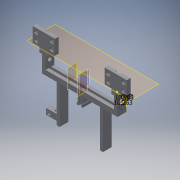
# Autodesk Inventor part: frontChassis_final
Saved by Autodesk Inventor 2018 (Build 220112000, 112)
## iProperties
Created: 2017-10-21
Part Number: frontChassis_final
Material: Generic
Document SubType Name: Modeling
Designer: Prakash
Density: 1 g/cm^3
Appearance: Default
d0: 1.500 mm
d1: 10.000 mm
d2: 18.000 mm
d3: 18.000 mm
d4: 30.000 mm
d5: 0.00 deg
d8: 10.000 mm
d9: 0.00 deg
d10: 3.588 mm
d11: 3.588 mm
d12: 34.763 mm
d13: 0.00 deg
d15: 9.763 mm
d16: 9.525 mm
d17: 8.000 mm
d19: 0.00 deg
d20: 4.000 mm
d21: 0.00 deg
d22: 10.000 mm
d25: 10.000 mm
d26: 5.000 mm
d27: 70.000 mm
d28: 0.00 deg
d74: 7.000 mm
d75: 7.000 mm
d76: 7.500 mm
d77: 7.500 mm
d79: 7.500 mm
d80: 7.500 mm
d81: 3.500 mm
d89: 8.000 mm
d90: 3.175 mm
d91: 0.00 deg
d104: -68.000 mm
d106: 19.526 mm
d107: 9.526 mm
d108: 8.000 mm
d112: 25.000 mm
d113: 7.175 mm
d114: 0.00 deg
d115: 4.000 mm
d116: 0.00 deg
d117: 45.250 mm
Author: Prakash
Autodesk Inventor part; units mm, degrees
ref_plane "YZ Plane" through (0, 0, 0) normal (1, 0, 0) x (0, 1, 0)
ref_plane "XZ Plane" through (0, 0, 0) normal (0, 1, 0) x (-1, 0, 0)
ref_plane "XY Plane" through (0, 0, 0) normal (0, 0, 1) x (1, 0, 0)
sketch "Sketch1" plane through (0, 0, 0) normal (0, 0, 1) x (1, 0, 0)
  line L0 (0, 0) -> (45.5394, 0)
  line L1 (45.5394, 0) -> (45.5394, 7.5)
  line L2 (45.5394, 7.5) -> (27.5394, 7.5)
  line L3 (0, 7.5) -> (0, 0)
  line L4 (22.7697, 7.5) -> (22.7697, 9) construction
  arc A0 (18, 7.5) -> (27.5394, 7.5) centre (22.7697, 9) ccw
  circle A1 centre (22.7697, 9) radius 9 construction
  line L5 (18, 7.5) -> (0, 7.5)
  line L6 (27.5394, 7.5) -> (22.7697, 7.5) construction
  line L7 (22.7697, 7.5) -> (18, 7.5) construction
  dimension "d0" = 1.5
  dimension "d1" = 10
  dimension "d2" = 18
  dimension "d3" = 18
  constraints: 16 end point, 5 parallel, 2 centre point, 2 coincident, 2 point on circle, 1 collinear, 1 horizontal, 1 perpendicular, 1 tangent, 1 vertical
  measures "d0" distance of L4.start L4.end
  measures "d1" diameter of A0
  measures "d2" distance of L1.end L2.end
  measures "d3" diameter of A1
extrude "Extrusion1" add sketch "Sketch1" along normal blind 30
sketch "Sketch3" plane through (0, 0, 0) normal (0, 0, -1) x (-1, 0, 0)
  circle A0 centre (-22.7697, 9) radius 9 construction
  arc A1 (-27.5394, 7.5) -> (-18, 7.5) centre (-22.7697, 9) ccw projected
  arc A2 (-27.5394, 7.5) -> (-18, 7.5) centre (-22.7697, 9) ccw projected
  arc A3 (-27.5394, 7.5) -> (-18, 7.5) centre (-22.7697, 9) ccw projected
  circle A4 centre (-22.7697, 9) radius 5
  line L0 (-31.7697, 9) -> (-31.7697, 0)
  line L1 (-13.7697, 9) -> (-13.7697, 0)
  arc A5 (-22.7697, 0) -> (-13.7697, 9) centre (-22.7697, 9) ccw
  line L2 (0, 0) -> (-45.5394, 0) projected
  line L3 (-31.7697, 0) -> (-22.7697, 0)
  line L4 (-22.7697, 0) -> (-13.7697, 0)
  arc A6 (-31.7697, 9) -> (-22.7697, 0) centre (-22.7697, 9) ccw
  arc A7 (-13.7697, 9) -> (-31.7697, 9) centre (-22.7697, 9) ccw
  constraints: 8 end point, 8 point on circle, 3 centre point, 2 coincident, 2 collinear, 2 point on line, 2 tangent, 2 vertical, 1 concentric, 3 other
extrude "Extrusion2" add sketch "Sketch3" along normal blind 10
sketch "Sketch5" plane through (0, 0, -10) normal (0, 0, -1) x (-1, 0, 0)
  line L0 (-31.7697, 0) -> (-13.7697, 0) projected
  line L1 (-22.7697, 0) -> (-19.1822, 0)
  line L2 (-22.7697, 0) -> (-26.3572, 0)
  line L3 (-26.3572, 0) -> (-19.1822, 0)
  line L4 (-19.1822, 0) -> (-19.1822, 18)
  line L5 (-19.1822, 18) -> (-26.3572, 18)
  line L6 (-26.3572, 18) -> (-26.3572, 0)
  arc A0 (-13.7697, 9) -> (-31.7697, 9) centre (-22.7697, 9) ccw projected
  point P0 (0, 0)
  dimension "d10" = 3.5875
  dimension "d11" = 3.5875
  constraints: 12 end point, 2 parallel, 2 point on line, 1 horizontal, 1 midpoint, 1 perpendicular, 1 tangent
  measures "d10" distance of L1.start L1.end
  measures "d11" distance of L1.start L2.end
extrude "Extrusion3" add sketch "Sketch5" along normal blind 34.763
sketch "Sketch6" plane through (26.3572, 5.5172, -10) normal (1, 0, 0) x (0, 0, -1)
  line L0 (-10, 3.4828) -> (0, 3.4828) projected
  line L1 (0, 3.4828) -> (9.763, 3.4828) construction
  circle A0 centre (9.763, 3.4828) radius 4.7625
  circle A1 centre (9.763, 3.4828) radius 4
  point P0 (-10, -5.5172)
  dimension "d15" = 9.763
  dimension "d16" = 9.525
  dimension "d17" = 8
  constraints: 2 centre point, 2 coincident, 2 end point, 1 horizontal
  measures "d15" distance of L0.end L1.end
  measures "d16" diameter of A0
  measures "d17" diameter of A1
extrude "Extrusion4" cut sketch "Sketch6" against normal up to next contours A0 | A1
sketch "Sketch7" plane through (19.1822, 5.5172, -10) normal (-1, 0, 0) x (0, 0, 1)
  circle A0 centre (-9.763, 3.4828) radius 4 projected
  circle A1 centre (-9.763, 3.4828) radius 4.7625 projected
  point P0 (10, -5.5172)
extrude "Extrusion5" add sketch "Sketch7" against normal blind 4
sketch "Sketch8" plane through (19.1822, 5.5172, -10) normal (-1, 0, 0) x (0, 0, 1)
  line L0 (-34.763, -5.5172) -> (-34.763, 12.4828) projected
  line L1 (-34.763, 12.4828) -> (-24.763, 12.4828)
  line L2 (-24.763, 12.4828) -> (-24.763, 5.9828)
  line L3 (-24.763, 5.9828) -> (-34.763, 5.9828)
  line L4 (-34.763, 5.9828) -> (-34.763, 12.4828)
  line L5 (-34.763, -5.5172) -> (-24.763, -5.5172)
  line L6 (-24.763, -5.5172) -> (-24.763, 0.9828)
  line L7 (-24.763, 0.9828) -> (-34.763, 0.9828)
  line L8 (-34.763, 0.9828) -> (-34.763, -5.5172)
  point P0 (10, -5.5172)
  dimension "d22" = 10
  dimension "d25" = 10
  dimension "d26" = 5
  constraints: 16 end point, 4 parallel, 2 horizontal, 2 perpendicular, 1 collinear
  measures "d22" distance of L2.end L3.end
  measures "d25" distance of L6.end L7.end
  measures "d26" distance between parallel lines of L7 L3
extrude "Extrusion6" add sketch "Sketch8" along normal blind 70
sketch "Sketch11" plane through (0, 7.5, 30) normal (0, 1, 0) x (1, 0, 0)
  line L0 (13.7697, 30) -> (0, 30) projected
  line L1 (7, 30) -> (7, 0)
  line L2 (18, 0) -> (0, 0) projected
  line L3 (38.5394, 30) -> (38.5394, 0)
  line L4 (0, 30) -> (0, 0) projected
  line L5 (45.5394, 30) -> (45.5394, 0) projected
  line L6 (45.5394, 30) -> (31.7697, 30) projected
  line L7 (45.5394, 0) -> (27.5394, 0) projected
  point P0 (7, 22.5)
  point P1 (7, 7.5)
  point P2 (38.5394, 22.5)
  point P3 (38.5394, 7.5)
  dimension "d74" = 7
  dimension "d75" = 7
  dimension "d76" = 7.5
  dimension "d77" = 7.5
  dimension "d79" = 7.5
  dimension "d80" = 7.5
  constraints: 8 point on line, 4 end point, 2 vertical
  measures "d74" distance between parallel lines of L4 L1
  measures "d75" distance between parallel lines of L5 L3
  measures "d76" distance of L1.start point (7, 22.5)
  measures "d77" distance of L1.end point (7, 7.5)
  measures "d79" distance of L3.start point (38.539, 22.5)
  measures "d80" distance of L3.end point (38.539, 7.5)
hole "Hole3" at (7, 7.5, 7.5) at (7, 7.5, 22.5) at (38.5394, 7.5, 7.5) at (38.5394, 7.5, 22.5) direction (0, -1, 0) diameter 3.5 end up to face face through (19.7697, 0, 20) facing (0, -1, 0)
sketch "Sketch13" plane through (0, 0, 30) normal (0, -1, 0) x (1, 0, 0)
  circle A0 centre (7, -7.5) radius 1.75 projected
  circle A1 centre (38.5394, -7.5) radius 1.75 projected
  circle A2 centre (38.5394, -22.5) radius 1.75 projected
  circle A3 centre (7, -22.5) radius 1.75 projected
  line L0 (11, -9.8094) -> (7, -12.1188)
  line L1 (7, -12.1188) -> (3, -9.8094)
  line L2 (3, -9.8094) -> (3, -5.1906)
  line L3 (3, -5.1906) -> (7, -2.8812)
  line L4 (7, -2.8812) -> (11, -5.1906)
  line L5 (11, -5.1906) -> (11, -9.8094)
  line L6 (11, -20.1906) -> (11, -24.8094)
  line L7 (11, -24.8094) -> (7, -27.1188)
  line L8 (7, -27.1188) -> (3, -24.8094)
  line L9 (3, -24.8094) -> (3, -20.1906)
  line L10 (3, -20.1906) -> (7, -17.8812)
  line L11 (7, -17.8812) -> (11, -20.1906)
  line L12 (42.5394, -20.1906) -> (42.5394, -24.8094)
  line L13 (42.5394, -24.8094) -> (38.5394, -27.1188)
  line L14 (38.5394, -27.1188) -> (34.5394, -24.8094)
  line L15 (34.5394, -24.8094) -> (34.5394, -20.1906)
  line L16 (34.5394, -20.1906) -> (38.5394, -17.8812)
  line L17 (38.5394, -17.8812) -> (42.5394, -20.1906)
  line L18 (38.5394, -2.8812) -> (42.5394, -5.1906)
  line L19 (42.5394, -5.1906) -> (42.5394, -9.8094)
  line L20 (42.5394, -9.8094) -> (38.5394, -12.1188)
  line L21 (38.5394, -12.1188) -> (34.5394, -9.8094)
  line L22 (34.5394, -9.8094) -> (34.5394, -5.1906)
  line L23 (34.5394, -5.1906) -> (38.5394, -2.8812)
  line L24 (0, -30) -> (0, 0) projected
  line L25 (45.5394, -30) -> (45.5394, 0) projected
  point P0 (38.5394, -22.5)
  point P1 (38.5394, -7.5)
  dimension "d89" = 8
  constraints: 48 end point, 4 coincident, 4 parallel, 3 equal length, 52 other
  measures "d89" distance between parallel lines of L0 L3
extrude "Extrusion7" cut sketch "Sketch13" against normal blind 3.175
mirror "Mirror1" about plane through (-50.8178, 14.75, -39.763) normal (-1, 0, 0) of "Extrusion6", "Extrusion3", "Extrusion5", "Extrusion4", "Extrusion2", "Extrusion1", "Hole3", "Extrusion7"
ref_plane "Work Plane1" through (-41.6428, 5.5172, -10) normal (1, 0, 0) x (0, 0, -1)
sketch "Sketch19" plane through (-41.6428, 5.5172, -10) normal (1, 0, 0) x (0, 0, -1)
  line L0 (0, 12.4828) -> (34.763, 12.4828) projected
  line L1 (0, 12.4828) -> (24.763, 12.4828) projected
  line L2 (24.763, 12.4828) -> (34.763, 12.4828)
  circle A0 centre (29.763, 37.4828) radius 9.763
  circle A1 centre (29.763, 37.4828) radius 4.763
  circle A2 centre (29.763, 37.4828) radius 4
  line L3 (34.763, 12.4828) -> (34.763, 29.0973)
  line L4 (24.763, 29.0973) -> (24.763, 12.4828)
  line L5 (29.763, 12.4828) -> (29.763, 37.4828) construction
  point P0 (-10, -5.5172)
  dimension "d106" = 19.526
  dimension "d107" = 9.526
  dimension "d108" = 8
  dimension "d112" = 25
  constraints: 8 end point, 3 centre point, 3 coincident, 2 perpendicular, 2 point on circle, 1 horizontal, 1 midpoint, 1 parallel
  measures "d106" diameter of A0
  measures "d107" diameter of A1
  measures "d108" diameter of A2
  measures "d112" distance from line of A0.centre L0
extrude "Extrusion10" add sketch "Sketch19" along normal blind 7.175 contours L4 A0 L3 L0 | A0
sketch "Sketch22" plane through (-41.6428, 5.5172, -10) normal (-1, 0, 0) x (0, 0, 1)
  circle A0 centre (-29.763, 37.4828) radius 4 projected
  circle A1 centre (-29.763, 37.4828) radius 4.763 projected
  point P0 (10, -5.5172)
extrude "Extrusion11" [suppressed]
ref_plane "Work Plane2" through (-75.5678, 5.5172, -10) normal (1, 0, 0) x (0, 0, -1)
mirror "Mirror2" [suppressed]
ref_plane "Work Plane4" through (-133.4053, 9, 0) normal (0, 0, 1) x (1, 0, 0)
split body "Split1" result two bodies by plane through (-133.4053, 9, 0) normal (0, 0, 1) first body at (-120.4821, 0.5, 13.2698) (18.8465, 0.5, 16.7302)
ref_plane "Halfway plane" through (-50.8178, 5.5172, -10) normal (-1, 0, 0) x (0, 0, 1)
sketch "Sketch23" plane through (-41.6428, 18, -34.763) normal (0, 1, 0) x (1, 0, 0)
  line L0 (68, 10) -> (-86.35, 10) construction
  line L1 (-9.175, 10) -> (-7.675, 10) construction
  line L2 (-9.175, 10) -> (-9.175, 27.798) construction
  arc A0 (-7.675, 21.7307) -> (-3.1077, 29.298) centre (-9.175, 27.798) ccw
  line L3 (-7.675, 10) -> (-4.675, 10)
  line L4 (-4.675, 10) -> (-4.675, 25.0565)
  line L5 (-4.675, 25.0565) -> (-7.675, 25.0565)
  line L6 (-7.675, 25.0565) -> (-7.675, 10)
  arc A1 (-7.675, 25.0565) -> (-6.4335, 29.298) centre (-9.175, 27.798) ccw
  line L7 (-6.4335, 29.298) -> (-3.1077, 29.298)
  point P0 (41.6428, -34.763)
  dimension "d119" = 1.5
  dimension "d120" = 17.798
  dimension "d121" = 12.5
  dimension "d122" = 3
  dimension "d123" = 6.25
  dimension "d125" = 19.298
  constraints: 14 end point, 4 point on circle, 2 centre point, 2 coincident, 2 horizontal, 2 parallel, 2 perpendicular, 2 point on line, 1 midpoint
  measures "d119" distance of L1.start L1.end
  measures "d120" distance of L1.start L2.end
  measures "d121" diameter of A0
  measures "d122" distance of L5.end L4.end
  measures "d123" diameter of A1
  measures "d125" distance between parallel lines of L0 L7
extrude "Extrusion12" add sketch "Sketch23" against normal blind 18 bodies 3
sketch "Sketch24" plane through (-46.3178, 18, -44.763) normal (1, 0, 0) x (0, 0, -1)
  line L0 (0, -6.5) -> (0, -11.5) projected
  line L1 (0, -9) -> (13.4607, -9)
  line L2 (13.4607, 0) -> (13.4607, -18) projected
  point P0 (-44.763, -18)
  point P1 (6.7303, -9)
  constraints: 3 midpoint, 2 end point
hole "Hole4" at (-46.3178, 9, -51.4933) direction (-1, 0, 0) diameter 3.5 end up to face face through (-49.3178, 8.1667, -54.8007) facing (-1, 0, 0) bodies 3
sketch "Sketch25" plane through (19.1822, 18, -10) normal (0, 1, 0) x (1, 0, 0)
  line L0 (0, 34.763) -> (-140, 34.763) projected
  line L1 (-28.5, 34.763) -> (-22.5, 34.763)
  line L2 (-22.5, 34.763) -> (-22.5, 111.763)
  line L3 (-22.5, 111.763) -> (-28.5, 111.763)
  line L4 (-28.5, 111.763) -> (-28.5, 34.763)
  line L5 (-70, -70.3526) -> (-70, 142.1156) projected
  point P0 (-19.1822, -10)
  point P1 (-65.5, 34.763)
  dimension "d135" = 6
  dimension "d136" = 77
  dimension "d137" = 41.5
  constraints: 8 end point, 2 parallel, 1 horizontal, 1 perpendicular, 1 point on line
  measures "d135" distance of L3.end L2.end
  measures "d136" distance of L2.end L1.end
  measures "d137" distance between parallel lines of L5 L4
extrude "Extrusion13" add sketch "Sketch25" against normal up to surface (18 mm away) bodies 3
mirror "Mirror3" about plane through (-50.8178, 5.5172, -10) normal (-1, 0, 0) of "Extrusion12", "Hole4", "Extrusion13" bodies 3
sketch "Sketch27" plane through (-127.9928, 18, -10) normal (0, 1, 0) x (1, 0, 0)
  line L0 (93.525, 20) -> (93.525, 39.526) projected
  line L1 (86.35, 20) -> (86.35, 39.526) projected
  line L2 (93.525, 39.526) -> (86.35, 39.526)
  line L3 (86.35, 39.526) -> (86.35, 20)
  line L4 (86.35, 20) -> (93.525, 20)
  line L5 (93.525, 20) -> (93.525, 39.526)
  point P0 (127.9928, -10)
  point P1 (93.525, 34.763)
  point P2 (93.525, 24.763)
  point P3 (86.35, 34.763)
  point P4 (86.35, 24.763)
  constraints: 8 end point, 2 parallel, 1 horizontal, 1 perpendicular
extrude "Extrusion14" cut sketch "Sketch27" along normal blind 42 bodies 3
sketch "Sketch28" plane through (-98.3178, 18, -121.763) normal (-1, 0, 0) x (0, 0, 1)
  line L0 (0, 0) -> (77, 0) projected
  line L1 (0, 0) -> (12, 0)
  line L2 (12, 0) -> (12, -10)
  line L3 (12, -10) -> (0, -10)
  line L4 (0, -10) -> (0, 0)
  point P0 (121.763, -18)
  dimension "d144" = 12
  dimension "d145" = 10
  constraints: 8 end point, 2 parallel, 1 horizontal, 1 perpendicular
  measures "d144" distance of L2.end L3.end
  measures "d145" distance of L1.end L2.end
extrude "Extrusion15" add sketch "Sketch28" along normal blind 30 bodies 3
sketch "Sketch29" plane through (26.3572, 18, -10) normal (0, 1, 0) x (1, 0, 0)
  line L0 (-118.675, 111.763) -> (-154.675, 111.763) projected
  line L1 (-124.675, 99.763) -> (-154.675, 99.763) projected
  line L2 (-154.675, 111.763) -> (-124.675, 111.763)
  line L3 (-124.675, 111.763) -> (-124.675, 99.763)
  line L4 (-124.675, 99.763) -> (-154.675, 99.763)
  line L5 (-154.675, 99.763) -> (-154.675, 111.763)
  line L6 (-124.675, 105.763) -> (-130.175, 105.763)
  line L7 (-154.675, 105.763) -> (-149.175, 105.763)
  point P0 (-26.3572, -10)
  dimension "d148" = 30
  dimension "d149" = 5.5
  dimension "d150" = 5.5
  constraints: 12 end point, 3 horizontal, 2 coincident, 2 midpoint, 2 parallel, 1 perpendicular
  measures "d148" distance of L1.start L4.end
  measures "d149" distance of L6.start L6.end
  measures "d150" distance of L7.start L7.end
hole "Hole5" at (-103.8178, 18, -115.763) at (-122.8178, 18, -115.763) direction (0, -1, 0) diameter 3.5 end up to face face through (-108.3178, 8, -113.763) facing (0, -1, 0) bodies 3
sketch "Sketch30" plane through (-98.3178, 8, -121.763) normal (0, -1, 0) x (1, 0, 0)
  circle A0 centre (-24.5, 6) radius 1.75 projected
  circle A1 centre (-5.5, 6) radius 1.75 projected
  circle A2 centre (-24.5, 6) radius 1.75 projected
  line L0 (-19.8812, 6) -> (-22.1906, 2)
  line L1 (-22.1906, 2) -> (-26.8094, 2)
  line L2 (-26.8094, 2) -> (-29.1188, 6)
  line L3 (-29.1188, 6) -> (-26.8094, 10)
  line L4 (-26.8094, 10) -> (-22.1906, 10)
  line L5 (-22.1906, 10) -> (-19.8812, 6)
  line L6 (-0.8812, 6) -> (-3.1906, 2)
  line L7 (-3.1906, 2) -> (-7.8094, 2)
  line L8 (-7.8094, 2) -> (-10.1188, 6)
  line L9 (-10.1188, 6) -> (-7.8094, 10)
  line L10 (-7.8094, 10) -> (-3.1906, 10)
  line L11 (-3.1906, 10) -> (-0.8812, 6)
  point P0 (98.3178, 121.763)
  dimension "d158" = 8
  constraints: 24 end point, 2 coincident, 2 horizontal, 1 equal length, 26 other
  measures "d158" distance between parallel lines of L1 L4
extrude "Extrusion16" cut sketch "Sketch30" against normal blind 3.175 bodies 3
sketch "Sketch32" plane through (26.3572, 5.5172, -10) normal (1, 0, 0) x (0, 0, -1)
  circle A0 centre (9.763, 3.4828) radius 4.7625 projected
  line L0 (9.763, 3.4828) -> (9.763, 13.7458)
  line L1 (9.763, 13.7458) -> (14.763, 13.7458)
  line L2 (9.763, 13.7458) -> (4.763, 13.7458)
  line L3 (9.763, 13.7458) -> (9.763, 18.7458)
  line L4 (4.763, 13.7458) -> (4.763, 18.7458)
  line L5 (4.763, 18.7458) -> (9.763, 18.7458)
  line L6 (14.763, 18.7458) -> (14.763, 13.7458)
  line L7 (9.763, 18.7458) -> (14.763, 18.7458)
  line L8 (9.763, 3.4828) -> (20.026, 3.4828)
  line L9 (14.763, 13.7458) -> (14.763, 12.4828)
  line L10 (0, 12.4828) -> (24.763, 12.4828) projected
  line L11 (4.763, 13.7458) -> (4.763, 12.4828)
  point P0 (-10, -5.5172)
  dimension "d181" = 10.263
  dimension "d182" = 5
  dimension "d183" = 5
  dimension "d184" = 5
  dimension "d185" = 10.263
  constraints: 22 end point, 4 vertical, 3 coincident, 3 horizontal, 3 perpendicular, 3 point on line, 1 parallel
  measures "d181" distance of L0.start L0.end
  measures "d182" distance of L0.end L1.end
  measures "d183" distance of L0.end L2.end
  measures "d184" distance of L0.end L3.end
  measures "d185" distance of L0.start L8.end
extrude "Extrusion18" add sketch "Sketch32" against normal up to surface (7.175 mm away) contours L10 L11 L2 L0 | L0 L1 L9 L10 | L3 L7 L6 L1 | L2 L4 L5 L3 bodies 3
hole "Hole7" at (26.3572, 19.263, -19.763) at (26.3572, 9, -30.026) direction (-1, 0, 0) diameter 3.5 end up to face face through (19.1822, 1.6764, -21.6694) facing (-1, 0, 0) bodies 3
ref_plane "Work Plane3" through (-109.4928, 5.5172, -10) normal (1, 0, 0) x (0, 0, -1)
equation "\"d183\" = d182"
equation "\"d184\" = d182"
body "Solid2"
body "Solid3"
